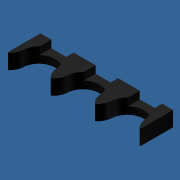
# Autodesk Inventor part: swirvy
Saved by Autodesk Inventor 2012 (Build 160160000, 160)
## iProperties
Created: 2012-02-03
Part Number: swirvy
Material: Default
Document SubType Name: Modeling
Designer: Allison Garza
Density: 1 g/cm^3
Author: Allison Garza
Autodesk Inventor part; units mm, degrees
ref_plane "YZ Plane" through (0, 0, 0) normal (1, 0, 0) x (0, 1, 0)
ref_plane "XZ Plane" through (0, 0, 0) normal (0, 1, 0) x (-1, 0, 0)
ref_plane "XY Plane" through (0, 0, 0) normal (0, 0, 1) x (1, 0, 0)
sketch "Sketch1" plane through (0, 0, 0) normal (0, 0, 1) x (1, 0, 0)
  line L0 (-32.1306, 17.7406) -> (444.1194, 17.7406)
  line L1 (444.1194, 17.7406) -> (444.1194, -33.0594)
  line L2 (444.1194, -33.0594) -> (-32.1306, -33.0594)
  line L3 (-32.1306, -33.0594) -> (-32.1306, 17.7406)
  point P0 (0, 0)
  dimension "d0" = 476.25
  dimension "d1" = 50.8
  constraints: 8 end point, 2 parallel, 1 horizontal, 1 perpendicular
  measures "d0" distance of L0.start L0.end
  measures "d1" distance of L2.end L0.start
extrude "Extrusion1" add sketch "Sketch1" along normal blind 139.7
sketch "Sketch2" plane through (-32.1306, 17.7406, 0) normal (0, 1, 0) x (1, 0, 0)
  line L0 (0, -139.7) -> (476.25, -139.7) projected
  line L1 (0, 0) -> (476.25, 0) projected
  line L2 (0, 0) -> (0, -139.7) projected
  circle A0 centre (75.1417, -80.645) radius 55.88
  circle A1 centre (225.4419, -80.645) radius 55.88
  circle A2 centre (375.7337, -80.645) radius 55.88
  line L3 (150.2833, 0) -> (150.2833, -139.7)
  line L4 (300.5751, 0) -> (300.5751, -139.7)
  line L5 (450.8669, 0) -> (450.8669, -139.7)
  arc A3 (131.0217, -80.645) -> (150.2833, -114.7129) centre (183.3802, -73.521) ccw
  arc A4 (150.2833, -114.7129) -> (169.5619, -80.645) centre (117.2054, -73.5058) ccw
  arc A5 (281.208, -77.0792) -> (300.5751, -114.6812) centre (333.9413, -73.7073) ccw
  arc A6 (300.5751, -114.6812) -> (319.9683, -77.068) centre (267.2357, -73.6855) ccw
  arc A7 (0, -114.6812) -> (19.2617, -80.645) centre (-33.0921, -73.4855) ccw
  arc A8 (431.6137, -80.645) -> (450.8669, -113.4262) centre (483.7537, -72.0665) ccw
  line L6 (450.8669, 0) -> (476.25, 0)
  line L7 (476.25, 0) -> (476.25, -139.7)
  line L8 (476.25, -139.7) -> (450.8669, -139.7)
  line L9 (450.8669, -139.7) -> (450.8669, 0)
  point P0 (32.1306, 0)
  dimension "d4" = 111.76
  dimension "d5" = 111.76
  dimension "d6" = 111.76
  dimension "d7" = 150.2833
  dimension "d8" = 150.2918
  dimension "d9" = 150.2918
  dimension "d10" = 75.1417
  dimension "d11" = 75.1332
  dimension "d12" = 75.1332
  dimension "d13" = 59.055
  constraints: 18 point on circle, 14 end point, 10 point on line, 9 centre point, 5 equal radius, 4 perpendicular, 2 horizontal alignment, 2 parallel, 2 tangent, 1 horizontal
  measures "d4" diameter of A0
  measures "d5" diameter of A1
  measures "d6" diameter of A2
  measures "d7" distance of L0.start L3.end
  measures "d8" distance of L3.end L4.end
  measures "d9" distance of L4.end L5.end
  measures "d10" horizontal distance of A0.centre L3.end
  measures "d11" horizontal distance of L4.end A1.centre
  measures "d12" horizontal distance of A2.centre L5.end
  measures "d13" vertical distance of L0.start A0.centre
extrude "Extrusion2" cut sketch "Sketch2" against normal blind 139.7 contours L2 A7 A0 A3 L3 L0 | L3 A4 A1 A5 L4 L0 | L4 A6 A2 A8 L5 L0 | A0 | L5 L1 L7 L0 | A1 | A2
fillet "Fillet1" radius 2.54 1 edges at (418.7363, -7.6594, 113.4262)
fillet "Fillet2" radius 2.54 1 edges at (268.4445, -7.6594, 114.6812)
fillet "Fillet3" radius 2.54 1 edges at (118.1527, -7.6594, 114.7129)
fillet "Fillet4" radius 2.54 1 edges at (-32.1306, -7.6594, 114.6812)
sketch "Sketch3" plane through (-32.1306, 17.7406, 0) normal (0, 1, 0) x (1, 0, 0)
  arc A0 (148.6129, -113.313) -> (151.9544, -113.3138) centre (150.2841, -111.4003) ccw projected
  arc A1 (298.8914, -113.2506) -> (302.2598, -113.2517) centre (300.5762, -111.3498) ccw projected
  line L0 (0, 0) -> (450.8669, 0) projected
  line L1 (37.0382, 0) -> (113.2382, 0)
  line L2 (113.2382, 0) -> (113.2382, -50.8)
  line L3 (113.2382, -50.8) -> (37.0382, -50.8)
  line L4 (37.0382, -50.8) -> (37.0382, 0)
  line L5 (150.2841, -111.4003) -> (150.2841, 5.0811)
  line L6 (263.53, 0) -> (187.33, 0)
  line L7 (187.33, 0) -> (187.33, -50.8)
  line L8 (187.33, -50.8) -> (263.53, -50.8)
  line L9 (263.53, -50.8) -> (263.53, 0)
  line L10 (75.1382, -50.8) -> (75.1382, 0)
  line L11 (300.5762, -111.3498) -> (300.5762, 0)
  line L12 (337.6224, -50.8) -> (337.6224, 0)
  line L13 (337.6224, 0) -> (413.8224, 0)
  line L14 (413.8224, 0) -> (413.8224, -50.8)
  line L15 (413.8224, -50.8) -> (337.6224, -50.8)
  point P0 (32.1306, 0)
  dimension "d20" = 76.2
  dimension "d21" = 50.8
  dimension "d22" = 0
  dimension "d23" = 38.1
  dimension "d24" = 75.1459
  constraints: 30 end point, 8 symmetric about line, 4 perpendicular, 2 midpoint, 2 parallel, 1 horizontal, 1 point on line
  measures "d20" distance of L1.start L1.end
  measures "d21" distance of L3.end L1.start
  measures "d22" vertical distance of L0.start L1.start
  measures "d23" distance between parallel lines of L2 L10
  measures "d24" distance between parallel lines of L5 L10
extrude "Extrusion3" cut sketch "Sketch3" against normal blind 25.4
body "Solid1"
